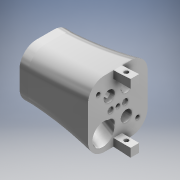
# Autodesk Inventor part: AA037
Saved by Autodesk Inventor 2017 SP1 (Build 210196100, 196)
## iProperties
Created: 2017-10-30
Part Number: AA037
Material: ABS Plastic
Document SubType Name: Modeling
Designer: Zach
Density: 1.06 g/cm^3
Appearance: CR White
Author: Zach
Autodesk Inventor part; units mm, degrees
ref_plane "YZ Plane" through (0, 0, 0) normal (1, 0, 0) x (0, 1, 0)
ref_plane "XZ Plane" through (0, 0, 0) normal (0, 1, 0) x (-1, 0, 0)
sketch "Sketch1" plane through (0, 0, 0) normal (0, 0, 1) x (1, 0, 0)
  line L0 (0, 0) -> (0, 60)
  line L1 (75, -8.75) -> (75, 68.75)
  arc A0 (0, 60) -> (75, 68.75) centre (-20.2749, 559.5888) ccw
  arc A1 (75, -8.75) -> (0, 0) centre (-20.2749, -499.5888) ccw
  point P0 (75, 30)
  point P1 (0, 30)
  dimension "d0" = 60
  dimension "d1" = 77.5
  dimension "d2" = 500
  dimension "d3" = 500
  dimension "d4" = 75
  constraints: 4 end point, 4 point on circle, 2 centre point, 2 midpoint, 2 vertical, 1 horizontal alignment
  measures "d0" distance of L0.start L0.end
  measures "d1" distance of L1.start L1.end
  measures "d2" radius of A0
  measures "d3" radius of A1
  measures "d4" distance between parallel lines of L1 L0
extrude "Extrusion1" add sketch "Sketch1" along normal blind 60
sketch "Sketch3" plane through (0, 0, 0) normal (0, 1, 0) x (-1, 0, 0)
  line L0 (-75, 65) -> (-75, -5) construction
  line L1 (-75, 0) -> (-75, 60) construction
  arc A0 (0, 0) -> (-75, -5) centre (28.972, -999.5802) ccw
  arc A1 (-75, 65) -> (0, 60) centre (28.972, 1059.5802) ccw
  line L2 (-75, 65) -> (-75, 60)
  line L3 (-75, 60) -> (0, 60) projected
  line L4 (-75, 60) -> (0, 60)
  line L5 (0, 0) -> (-75, 0) projected
  line L6 (0, 0) -> (-75, 0)
  line L7 (-75, 0) -> (-75, -5)
  point P0 (-75, 30)
  dimension "d10" = 70
  dimension "d11" = 1000
  dimension "d12" = 1000
  constraints: 10 end point, 4 point on circle, 2 centre point, 2 collinear, 2 horizontal, 2 midpoint, 1 horizontal alignment, 1 vertical, 1 vertical alignment
  measures "d10" distance of L0.start L0.end
  measures "d11" radius of A0
  measures "d12" radius of A1
extrude "Extrusion2" add sketch "Sketch3" along normal blind 75 and the other way blind 15
sketch "Sketch4" plane through (0, 75, 0) normal (0, 0, 1) x (1, 0, 0)
  arc A0 (0, -15) -> (75, -6.25) centre (-20.2749, 484.5888) ccw projected
  line L0 (75, -6.25) -> (75, 0) projected
  line L1 (0, 0) -> (75, 0) projected
  line L2 (0, 0) -> (0, -15) projected
  arc A1 (75, -83.75) -> (0, -75) centre (-20.2749, -574.5888) ccw projected
  line L3 (0, -75) -> (0, -90) projected
  line L4 (75, -90) -> (0, -90) projected
  line L5 (75, -90) -> (75, -83.75) projected
extrude "Extrusion3" cut sketch "Sketch4" along normal through all both and the other way through all
fillet "Fillet1" radius 20 4 edges at (37.9133, 62.9862, -1.8196) (37.9133, 62.9862, 61.8196) (37.9133, -2.9862, -1.8196) (37.9133, -2.9862, 61.8196)
sketch "Sketch5" plane through (0, 19.9929, 60) normal (-1, 0, 0) x (0, 0, 1)
  line L0 (-20, 25.0071) -> (-40, 25.0071) construction
  line L1 (-40, 25.0071) -> (-40, -4.9929) construction
  line L2 (-40, -4.9929) -> (-20, -4.9929) construction
  line L3 (-20, -4.9929) -> (-20, 25.0071) construction
  line L4 (0, 20.0142) -> (0, 0) projected
  line L5 (-40.0151, -19.9929) -> (-19.9849, -19.9929) projected
  circle A0 centre (-20, 25.0071) radius 2.5
  circle A1 centre (-20, -4.9929) radius 2.5
  circle A2 centre (-40, -4.9929) radius 2.5
  circle A3 centre (-40, 25.0071) radius 2.5
  circle A4 centre (-30, 10.0071) radius 13
  point P0 (-60, -19.9929)
  point P1 (-20, 10.0071)
  point P2 (0, 10.0071)
  point P3 (-30, -4.9929)
  point P4 (-30, -19.9929)
  point P5 (0, 10.0071)
  point P6 (-30, -19.9929)
  dimension "d20" = 20
  dimension "d21" = 30
  dimension "d22" = 5
  dimension "d23" = 5
  dimension "d24" = 5
  dimension "d25" = 5
  dimension "d26" = 26
  constraints: 8 end point, 6 midpoint, 5 centre point, 4 coincident, 2 horizontal alignment, 2 parallel, 2 vertical alignment, 1 horizontal, 1 perpendicular
  measures "d20" distance of L2.end L1.end
  measures "d21" distance of L1.end L0.end
  measures "d22" diameter of A0
  measures "d23" diameter of A1
  measures "d24" diameter of A2
  measures "d25" diameter of A3
  measures "d26" diameter of A4
extrude "Extrusion4" cut sketch "Sketch5" against normal through all
ref_plane "Work Plane1" through (5, 19.9929, 60) normal (-1, 0, 0) x (0, 0, 1)
sketch "Sketch7" plane through (5, 19.9929, 60) normal (-1, 0, 0) x (0, 0, 1)
  circle A0 centre (-40, 25.0071) radius 2.5 projected
  circle A1 centre (-20, 25.0071) radius 2.5 projected
  circle A2 centre (-20, -4.9929) radius 2.5 projected
  circle A3 centre (-40, -4.9929) radius 2.5 projected
  circle A4 centre (-40, 25.0071) radius 6.5
  circle A5 centre (-20, 25.0071) radius 6.5
  circle A6 centre (-20, -4.9929) radius 6.5
  circle A7 centre (-40, -4.9929) radius 6.5
  point P0 (-60, -19.9929)
  dimension "d38" = 13
  dimension "d39" = 13
  dimension "d40" = 13
  dimension "d41" = 13
  constraints: 4 centre point, 4 coincident
  measures "d38" diameter of A4
  measures "d39" diameter of A5
  measures "d40" diameter of A6
  measures "d41" diameter of A7
extrude "Extrusion6" cut sketch "Sketch7" against normal through all contours A0 | A1 | A2 | A3 | A4 | A5 | A6 | A7
sketch "Sketch9" plane through (75, 11.2166, -5) normal (1, 0, 0) x (0, 0, -1)
  circle A0 centre (-35, 18.7834) radius 2.5
  circle A1 centre (-26.5, 18.7834) radius 1.5
  circle A2 centre (-43.5, 18.7834) radius 1.5
  line L0 (-43.5, 18.7834) -> (-26.5, 18.7834) construction
  arc A3 (-25.1657, 27.2855) -> (-30.9343, 31.1313) centre (-35, 18.7834) ccw construction
  arc A4 (-30.9343, 6.4355) -> (-25.1657, 10.2813) centre (-35, 18.7834) ccw construction
  arc A5 (-44.8343, 10.2813) -> (-39.0657, 6.4355) centre (-35, 18.7834) ccw construction
  arc A6 (-39.0657, 6.4355) -> (-30.9343, 6.4355) centre (-35, 18.7834) ccw
  arc A7 (-25.1657, 10.2813) -> (-25.1657, 27.2855) centre (-35, 18.7834) ccw
  arc A8 (-30.9343, 31.1313) -> (-39.0657, 31.1313) centre (-35, 18.7834) ccw
  arc A9 (-30.9343, 31.1313) -> (-39.0657, 31.1313) centre (-35, 18.7834) ccw projected
  arc A10 (-44.8343, 27.2855) -> (-44.8343, 10.2813) centre (-35, 18.7834) ccw
  arc A11 (-44.8343, 27.2855) -> (-39.0657, 31.1313) centre (-45, 33.7834) ccw
  arc A12 (-25.1657, 10.2813) -> (-30.9343, 6.4355) centre (-25, 3.7834) ccw
  arc A13 (-39.0657, 6.4355) -> (-44.8343, 10.2813) centre (-45, 3.7834) ccw
  circle A14 centre (-45, 33.7834) radius 2.5 projected
  circle A15 centre (-45, 3.7834) radius 2.5 projected
  circle A16 centre (-25, 3.7834) radius 2.5 projected
  circle A17 centre (-25, 33.7834) radius 2.5 projected
  arc A18 (-30.9343, 31.1313) -> (-25.1657, 27.2855) centre (-25, 33.7834) ccw
  point P0 (-5, -11.2166)
  dimension "d47" = 5
  dimension "d48" = 3
  dimension "d49" = 3
  dimension "d50" = 17
  constraints: 16 point on circle, 14 centre point, 6 coincident, 4 concentric, 2 end point, 1 horizontal, 1 midpoint
  measures "d47" diameter of A0
  measures "d48" diameter of A1
  measures "d49" diameter of A2
  measures "d50" distance of L0.start L0.end
extrude "Extrusion8" add sketch "Sketch9" against normal blind 5 contours A13 A10 A11 A8 A18 A7 A12 A6
sketch "Sketch10" plane through (70, 11.2166, -5) normal (-1, 0, 0) x (0, 0, 1)
  circle A0 centre (35, 18.7834) radius 2.5 projected
  circle A1 centre (35, 18.7834) radius 4
  point P0 (5, -11.2166)
  dimension "d53" = 8
  constraints: 1 centre point, 1 coincident
  measures "d53" diameter of A1
extrude "Extrusion9" cut sketch "Sketch10" against normal blind 3
sketch "Sketch11" plane through (75, 11.2166, -5) normal (1, 0, 0) x (0, 0, -1)
  circle A0 centre (-43.5, 18.7834) radius 1.5 projected
  circle A1 centre (-26.5, 18.7834) radius 1.5 projected
  circle A2 centre (-26.5, 18.7834) radius 3.5
  circle A3 centre (-43.5, 18.7834) radius 3.5
  point P0 (-5, -11.2166)
  dimension "d56" = 7
  dimension "d57" = 7
  constraints: 2 centre point, 2 coincident
  measures "d56" diameter of A2
  measures "d57" diameter of A3
extrude "Extrusion10" cut sketch "Sketch11" against normal blind 3 contours A0 | A1 | A2 | A3
sketch "Sketch12" plane through (75, 11.2166, -5) normal (1, 0, 0) x (0, 0, -1)
  circle A0 centre (-57.981, 41.7644) radius 2.5
  circle A1 centre (-12.019, -4.1976) radius 2.5
  circle A2 centre (-35, 18.7834) radius 2.5 projected
  line L0 (-12.019, -4.1976) -> (-57.981, 41.7644) construction
  circle A3 centre (-35, 18.7834) radius 2.5 projected
  line L1 (-35, 18.7834) -> (-93.6923, 18.7834) construction
  point P0 (-5, -11.2166)
  dimension "d60" = 5
  dimension "d61" = 5
  dimension "d62" = 65
  dimension "d83" = 45
  constraints: 4 end point, 2 centre point, 1 coincident, 1 horizontal, 1 midpoint
  measures "d60" diameter of A0
  measures "d61" diameter of A1
  measures "d62" distance of L0.start L0.end
  measures "d83" angle of L0 L1
extrude "Extrusion11" cut sketch "Sketch12" against normal blind 25 contours A0 | A1
ref_plane "Work Plane2" through (75, 68.75, 30) normal (0, 0, 1) x (1, 0, 0)
sketch "Sketch13" plane through (75, 68.75, 30) normal (0, 0, 1) x (1, 0, 0)
  line L0 (20, 1.1827) -> (20, -8.8173)
  line L1 (20, -8.8173) -> (0, -8.8173)
  line L2 (20, -78.6827) -> (20, -68.6827)
  line L3 (20, -68.6827) -> (0, -68.6827)
  line L4 (0, -8.8173) -> (0, 0)
  line L5 (0, -77.5) -> (0, -68.6827)
  arc A0 (20, -78.6827) -> (0, -77.5) centre (-57.8838, -1226.0423) ccw
  arc A1 (0, 0) -> (20, 1.1827) centre (-57.8838, 1148.5423) ccw
  line L6 (95, 8.75) -> (95, -86.25) construction
  line L7 (0, -19.9666) -> (0, -57.5334) projected
  arc A2 (0, 0) -> (95, 8.75) centre (-57.8838, 1148.5423) ccw construction
  arc A3 (95, -86.25) -> (0, -77.5) centre (-57.8838, -1226.0423) ccw construction
  point P0 (-75, -68.75)
  point P1 (-75, -8.75)
  point P2 (0, -38.75)
  point P3 (95, -38.75)
  dimension "d67" = 20
  dimension "d68" = 10
  dimension "d69" = 10
  dimension "d75" = 1150
  dimension "d76" = 1150
  dimension "d77" = 95
  dimension "d78" = 95
  dimension "d79" = 1150
  dimension "d80" = 1150
  constraints: 14 end point, 10 point on circle, 4 centre point, 4 vertical, 2 midpoint, 2 perpendicular, 1 collinear, 1 horizontal alignment, 1 vertical alignment
  measures "d67" horizontal distance of L4.end L0.start
  measures "d68" distance of L0.start L0.end
  measures "d69" distance of L2.start L2.end
  measures "d75" radius of A0
  measures "d76" radius of A1
  measures "d77" distance of L6.start L6.end
  measures "d78" distance between parallel lines of L6 L7
  measures "d79" radius of A2
  measures "d80" radius of A3
extrude "Extrusion12" add sketch "Sketch13" along normal mid plane 10
sketch "Sketch14" plane through (75, 0.0673, 35) normal (0, 1, 0) x (1, 0, 0)
  circle A0 centre (10, 5) radius 2.5
  line L0 (20, 0) -> (20, 10) projected
  line L1 (0, 10) -> (20, 10) projected
  point P0 (-75, 35)
  point P1 (20, 5)
  dimension "d72" = 5
  dimension "d81" = 10
  constraints: 1 centre point, 1 horizontal alignment, 1 midpoint
  measures "d72" diameter of A0
  measures "d81" horizontal distance of L1.start A0.centre
extrude "Extrusion13" cut sketch "Sketch14" along normal through all both and the other way through all
sketch "Sketch17" plane through (0, 19.9929, 60) normal (-1, 0, 0) x (0, 0, 1)
  circle A0 centre (-40, 25.0071) radius 2.5 projected
  circle A1 centre (-20, -4.9929) radius 2.5 projected
  circle A2 centre (-20, 25.0071) radius 2.5 projected
  circle A3 centre (-40, -4.9929) radius 2.5 projected
  circle A4 centre (-30, 10.0071) radius 13 projected
  spline S0 degree 7 poles (0, 0) (0, -1.0232) (-0.061, -2.0684) (-0.1877, -3.13) (-0.3842, -4.2012) (-0.6535, -5.2742) (-0.997, -6.3404) (-1.8356, -8.4502) (-2.3318, -9.4935) (-2.9031, -10.512) (-3.5476, -11.4965) (-4.2617, -12.4381) (-5.0399, -13.3289) (-6.7073, -14.9914) (-7.596, -15.7638) (-8.535, -16.4724) (-9.5161, -17.1119) (-10.5308, -17.6787) (-11.5697, -18.171) (-13.6709, -19.0031) (-14.7328, -19.3441) (-15.8013, -19.6114) (-16.868, -19.8065) (-17.9251, -19.9323) (-18.9659, -19.9929) (-19.9849, -19.9929) knots 0 0 0 0 0 0 0 0 0.249525 0.249525 0.249525 0.249525 0.249525 0.249525 0.501026 0.501026 0.501026 0.501026 0.501026 0.501026 0.751429 0.751429 0.751429 0.751429 0.751429 0.751429 1 1 1 1 1 1 1 1 projected
  line L0 (0, 20.0142) -> (0, 0) projected
  spline S1 degree 7 poles (-19.9849, 40.0071) (-18.9661, 40.0071) (-17.9254, 39.9466) (-16.8684, 39.8208) (-15.8019, 39.6257) (-14.7336, 39.3585) (-13.6717, 39.0176) (-11.5706, 38.1856) (-10.5314, 37.6933) (-9.5167, 37.1264) (-8.5354, 36.4869) (-7.5963, 35.7782) (-6.7074, 35.0058) (-5.0399, 33.3431) (-4.2617, 32.4524) (-3.5476, 31.5107) (-2.9031, 30.5262) (-2.3318, 29.5077) (-1.8356, 28.4644) (-0.997, 26.3546) (-0.6535, 25.2884) (-0.3842, 24.2154) (-0.1877, 23.1442) (-0.061, 22.0826) (0, 21.0374) (0, 20.0142) knots 0 0 0 0 0 0 0 0 0.248536 0.248536 0.248536 0.248536 0.248536 0.248536 0.498974 0.498974 0.498974 0.498974 0.498974 0.498974 0.750475 0.750475 0.750475 0.750475 0.750475 0.750475 1 1 1 1 1 1 1 1 projected
  line L1 (-40.0151, 40.0071) -> (-19.9849, 40.0071) projected
  spline S2 degree 7 poles (-60, 20.0142) (-60, 21.0374) (-59.939, 22.0826) (-59.8123, 23.1442) (-59.6158, 24.2154) (-59.3465, 25.2884) (-59.003, 26.3546) (-58.1644, 28.4644) (-57.6682, 29.5077) (-57.0969, 30.5262) (-56.4524, 31.5107) (-55.7383, 32.4524) (-54.9601, 33.3431) (-53.2926, 35.0058) (-52.4037, 35.7782) (-51.4646, 36.4869) (-50.4833, 37.1264) (-49.4686, 37.6933) (-48.4294, 38.1856) (-46.3283, 39.0176) (-45.2664, 39.3585) (-44.1981, 39.6257) (-43.1316, 39.8208) (-42.0746, 39.9466) (-41.0339, 40.0071) (-40.0151, 40.0071) knots 0 0 0 0 0 0 0 0 0.249525 0.249525 0.249525 0.249525 0.249525 0.249525 0.501026 0.501026 0.501026 0.501026 0.501026 0.501026 0.751464 0.751464 0.751464 0.751464 0.751464 0.751464 1 1 1 1 1 1 1 1 projected
  line L2 (-60, 0) -> (-60, 20.0142) projected
  spline S3 degree 7 poles (-40.0151, -19.9929) (-41.0341, -19.9929) (-42.0749, -19.9323) (-43.132, -19.8065) (-44.1987, -19.6114) (-45.2672, -19.3441) (-46.3291, -19.0031) (-48.4303, -18.171) (-49.4692, -17.6787) (-50.4839, -17.1119) (-51.465, -16.4724) (-52.404, -15.7638) (-53.2927, -14.9914) (-54.9601, -13.3289) (-55.7383, -12.4381) (-56.4524, -11.4965) (-57.0969, -10.512) (-57.6682, -9.4935) (-58.1644, -8.4502) (-59.003, -6.3404) (-59.3465, -5.2742) (-59.6158, -4.2012) (-59.8123, -3.13) (-59.939, -2.0684) (-60, -1.0232) (-60, 0) knots 0 0 0 0 0 0 0 0 0.248571 0.248571 0.248571 0.248571 0.248571 0.248571 0.498974 0.498974 0.498974 0.498974 0.498974 0.498974 0.750475 0.750475 0.750475 0.750475 0.750475 0.750475 1 1 1 1 1 1 1 1 projected
  line L3 (-40.0151, -19.9929) -> (-19.9849, -19.9929) projected
  point P0 (-60, -19.9929)
  constraints: 4 other
extrude "Extrusion15" add sketch "Sketch17" along normal blind 10
ref_plane "Work Plane4" through (75, 11.2166, 65) normal (0.9526926, -0.2135155, 0.2163053) x (0, -0.7116813, -0.7025025)
sketch "Sketch16" plane through (75, 11.2166, 65) normal (0.9526926, -0.2135155, 0.2163053) x (0, -0.7116813, -0.7025025)
  circle A0 centre (13.6044, 11.4156) radius 12.5
  line L0 (13.6044, 11.4156) -> (11.2198, 36.3016) construction
  ellipse E0 centre (11.2198, 36.3016) end of major axis (8.7198, 36.3016) minor radius 2.3817 projected
  ellipse E1 centre (14.87, -1.7931) end of major axis (12.37, -1.7931) minor radius 2.3817 projected
  point P0 (65, -11.2166)
  dimension "d86" = 25
  dimension "d87" = 25
  constraints: 2 end point, 1 centre point, 1 coincident, 1 point on line, 2 other
  measures "d86" diameter of A0
  measures "d87" distance of L0.start L0.end
extrude "Extrusion14" cut sketch "Sketch16" along normal blind 5 and the other way blind 100 contours A0 E1 | E1 A0 picked at (13.8519, 16.0739) picked at (14.731, -0.4777)
equation "\"d3\" = d2"
equation "\"d23\" = d22"
equation "\"d24\" = d22"
equation "\"d25\" = d22"
body "Solid1"
